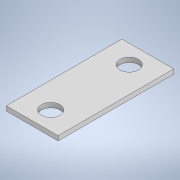
# Autodesk Inventor part: Adjustments
Saved by Autodesk Inventor 2022 (Build 260153000, 153)
## iProperties
Created: 2023-04-04
Part Number: Adjustments
Material: Generic
Document SubType Name: Modeling
Designer: zarek
Density: 1 g/cm^3
Appearance: Default
Author: zarek
Autodesk Inventor part; units mm, degrees
ref_plane "YZ Plane" through (0, 0, 0) normal (1, 0, 0) x (0, 1, 0)
ref_plane "XZ Plane" through (0, 0, 0) normal (0, 1, 0) x (-1, 0, 0)
ref_plane "XY Plane" through (0, 0, 0) normal (0, 0, 1) x (1, 0, 0)
sketch "Sketch1" plane through (0, 0, 0) normal (0, 1, 0) x (-1, 0, 0)
  line L0 (0, 0) -> (-11.2, 0)
  line L1 (-11.2, 0) -> (-11.2, -25)
  line L2 (-11.2, -25) -> (0, -25)
  line L3 (0, -25) -> (0, 0)
  circle A0 centre (-5.6, -4) radius 2
  circle A1 centre (-5.6, -21) radius 2
  dimension "d0" = 25
  dimension "d1" = 11.2
  dimension "d7" = 4
  dimension "d8" = 4
  dimension "d9" = 17
  dimension "d10" = 5.6
  dimension "d11" = 4
  dimension "d12" = 4
  constraints: 8 end point, 2 centre point, 2 parallel, 1 horizontal, 1 perpendicular
  measures "d0" distance of L1.end L0.end
  measures "d1" distance between parallel lines of L1 L3
  measures "d7" distance from line of L2 A1.centre
  measures "d8" distance from line of L0 A0.centre
  measures "d9" distance of A1.centre A0.centre
  measures "d10" distance from line of A1.centre L3
  measures "d11" diameter of A0
  measures "d12" diameter of A1
extrude "Extrusion1" add sketch "Sketch1" along normal blind 1
body "Solid1"
